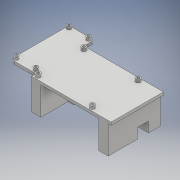
# Autodesk Inventor part: baseRaspberry
Saved by Autodesk Inventor 2018 (Build 220112000, 112)
## iProperties
Created: 2018-02-26
Part Number: baseRaspberry
Material: Genérico
Document SubType Name: Modeling
Designer: ivanb
Density: 1 g/cm^3
Appearance: Valor por defecto
Author: ivanb
## iProperties of the stored document baseRaspberry_3DPrint.ipt
Created: 2018-03-07
Part Number: baseRaspberry_3DPrint
Material: Genérico
Document SubType Name: Modeling
Designer: ivanb
Density: 1 g/cm^3
Appearance: Valor por defecto
Author: ivanb
Autodesk Inventor part; units mm, degrees
ref_plane "Plano de trabajo1" through (-77.1004, 28.9483, 0) normal (0, 0, -1) x (-1, 0, 0)
sketch "Boceto1" plane through (-77.1004, 28.9483, 0) normal (0, 0, -1) x (-1, 0, 0)
  line L0 (82, -56) -> (-3, -56)
  line L1 (-3, -56) -> (-3, 0)
  line L2 (-3, 0) -> (82, 0)
  line L3 (82, 0) -> (82, -56)
  point P0 (-77.1004, -28.9483)
  constraints: 8 end point, 2 parallel, 1 horizontal, 1 perpendicular
extrude "Extrusión1" add sketch "Boceto1" along normal blind 20
ref_plane "Plano de trabajo3" through (-77.1004, 28.9483, 0) normal (0, 0, 1) x (1, 0, 0)
sketch "Boceto2" plane through (-77.1004, 28.9483, 0) normal (0, 0, 1) x (1, 0, 0)
  circle A0 centre (-78.5, -3.5) radius 1.375 projected
  circle A1 centre (-78.5, -3.5) radius 1.125
  circle A2 centre (-20.5, -3.5) radius 1.375 projected
  circle A3 centre (-20.5, -3.5) radius 1.125
  circle A4 centre (-20.5, -52.5) radius 1.375 projected
  circle A5 centre (-20.5, -52.5) radius 1.125
  circle A6 centre (-78.5, -52.5) radius 1.375 projected
  circle A7 centre (-78.5, -52.5) radius 1.125
  line L0 (-91.1268, 5.8368) -> (25.5851, 5.8368)
  line L1 (25.5851, 5.8368) -> (25.5851, -70.6743)
  line L2 (25.5851, -70.6743) -> (-91.1268, -70.6743)
  line L3 (-91.1268, -70.6743) -> (-91.1268, 5.8368)
  point P0 (77.1004, -28.9483)
  dimension "d3" = 2.25
  dimension "d4" = 2.25
  dimension "d5" = 2.25
  dimension "d6" = 2.25
  constraints: 8 end point, 4 centre point, 4 coincident, 2 parallel, 1 horizontal, 1 perpendicular
  measures "d3" diameter of A1
  measures "d4" diameter of A3
  measures "d5" diameter of A5
  measures "d6" diameter of A7
extrude "Extrusión2" cut sketch "Boceto2" against normal blind 10 contours L0 L1 L2 L3
ref_plane "Plano de trabajo2" through (-77.1004, 28.9483, -20) normal (0, 0, -1) x (-1, 0, 0)
sketch "Boceto8" plane through (-77.1004, 28.9483, -20) normal (0, 0, -1) x (-1, 0, 0)
  circle A0 centre (77, -33) radius 1.25
  circle A1 centre (77, -5) radius 1.25
  line L0 (-3, -56) -> (82, -56) projected
  circle A2 centre (5, -33) radius 1.25
  circle A3 centre (5, -5) radius 1.25
  line L1 (82, -56) -> (82, 0) projected
  line L2 (82, -56) -> (72, -56)
  line L3 (72, -56) -> (72, 0)
  line L4 (72, 0) -> (82, 0)
  line L5 (82, 0) -> (82, -56)
  line L6 (10.1328, -56) -> (0.1328, -56)
  line L7 (5, -33) -> (5, -5)
  line L8 (0, -59.0097) -> (0, -32.6767)
  line L9 (79, -56) -> (0, -56) projected
  line L10 (0, -56) -> (10, -56)
  line L11 (10, -56) -> (10, 0)
  line L12 (10, 0) -> (0, 0)
  line L13 (0, 0) -> (0, -56)
  line L14 (82, 0) -> (-3, 0) projected
  point P0 (-77.1004, -28.9483)
  dimension "d31" = 2.5
  dimension "d32" = 2.5
  dimension "d33" = 28
  dimension "d35" = 2.5
  dimension "d36" = 72
  dimension "d37" = 2.5
  dimension "d38" = 5
  dimension "d39" = 72
  dimension "d40" = 5
  dimension "d41" = 28
  dimension "d43" = 10
  dimension "d45" = 5
  dimension "d46" = 10
  dimension "d92" = 0
  constraints: 22 end point, 4 centre point, 4 parallel, 3 horizontal, 2 perpendicular, 1 point on line, 1 vertical
  measures "d31" diameter of A0
  measures "d32" diameter of A1
  measures "d33" distance of A1.centre A0.centre
  measures "d35" diameter of A2
  measures "d36" distance of L7.start A0.centre
  measures "d37" diameter of A3
  measures "d38" distance from line of L1 A0.centre
  measures "d39" distance of L7.end A1.centre
  measures "d40" distance from line of L1 A1.centre
  measures "d41" distance of L7.end L7.start
  measures "d43" distance of L3.end L4.end
  measures "d45" distance from line of L7.start L8
  measures "d46" distance of L12.end L11.end
  measures "d92" distance between parallel lines of L14 L12
extrude "Extrusión8" add sketch "Boceto8" along normal blind 30 contours L8 L13 L12 L11 L0 | L3 L4 L1 L0
ref_plane "Plano de trabajo6" through (-159.1004, -27.0517, -10) normal (-1, 0, 0) x (0, 0, 1)
sketch "Boceto9" plane through (-159.1004, -27.0517, -10) normal (-1, 0, 0) x (0, 0, 1)
  line L0 (-29, 31) -> (-40, 31)
  line L1 (-40, 31) -> (-40, 43)
  line L2 (-40, 43) -> (-29, 43)
  line L3 (-29, 43) -> (-29, 31)
  line L4 (0, 0) -> (-40, 0) projected
  line L5 (-40, 0) -> (-40, 56) projected
  line L6 (0, 56) -> (-40, 56) projected
  point P0 (10, 27.0517)
  dimension "d49" = 11
  dimension "d50" = 12
  dimension "d52" = 0
  dimension "d82" = 13
  constraints: 8 end point, 2 parallel, 1 horizontal, 1 perpendicular
  measures "d49" distance of L1.end L2.end
  measures "d50" distance of L0.end L1.end
  measures "d52" distance between parallel lines of L5 L1
  measures "d82" distance between parallel lines of L6 L2
extrude "Extrusión9" cut sketch "Boceto9" against normal blind 100
ref_plane "Plano de trabajo5" through (-149.1004, -27.0517, -20) normal (1, 0, 0) x (0, 0, -1)
sketch "Boceto10" plane through (-149.1004, -27.0517, -20) normal (1, 0, 0) x (0, 0, -1)
  line L0 (17, 29) -> (30, 29)
  line L1 (30, 29) -> (30, 45)
  line L2 (30, 45) -> (17, 45)
  line L3 (17, 45) -> (17, 29)
  line L4 (-10, 56) -> (30, 56) projected
  line L5 (30, 31) -> (30, 0) projected
  line L6 (19, 31) -> (19, 43) projected
  line L7 (30, 31) -> (19, 31)
  line L8 (19, 31) -> (19, 43)
  line L9 (19, 43) -> (30, 43) projected
  line L10 (19, 43) -> (30, 43)
  point P0 (-20, 27.0517)
  dimension "d59" = 13
  dimension "d60" = 16
  constraints: 14 end point, 4 equal length, 2 perpendicular, 1 horizontal
  measures "d59" distance of L0.start L0.end
  measures "d60" distance of L0.end L1.end
extrude "Extrusión10" add sketch "Boceto10" along normal blind 6 contours L3 L2 L1 L9 L6 L7 L0
sketch "Boceto11" plane through (-77.1004, -27.0517, -20) normal (1, 0, 0) x (0, 0, -1)
  line L0 (30, 43) -> (30, 74)
  line L1 (17, 29) -> (30, 29)
  line L2 (30, 29) -> (30, 45)
  line L3 (30, 45) -> (17, 45)
  line L4 (17, 45) -> (17, 29)
  line L5 (30, 31) -> (19, 31)
  line L6 (19, 31) -> (30, 31)
  line L7 (30, 31) -> (19, 31)
  line L8 (19, 31) -> (19, 43)
  line L9 (19, 31) -> (19, 43)
  line L10 (30, 43) -> (19, 43)
  line L11 (19, 43) -> (30, 43)
  line L12 (19, 43) -> (30, 43) projected
  point P0 (-20, 27.0517)
  point P1 (-20, 27.0517)
  dimension "d64" = 13
  dimension "d65" = 16
  dimension "d66" = 2
  dimension "d88" = 0
  dimension "d89" = 2
  constraints: 24 end point, 3 equal length, 3 perpendicular, 1 horizontal, 1 point on line
  measures "d64" distance of L1.start L1.end
  measures "d65" distance of L1.end L2.end
  measures "d66" distance between parallel lines of L1 L5
  measures "d88" distance between parallel lines of L12 L10
  measures "d89" distance between parallel lines of L3 L10
extrude "Extrusión11" add sketch "Boceto11" against normal blind 16 contours L10 L8 L5 L2 L1 L4 L3 L0
ref_plane "Plano de trabajo4" through (-159.1004, -27.0517, -10) normal (0, -1, 0) x (1, 0, 0)
sketch "Boceto12" plane through (-159.1004, -27.0517, -10) normal (0, -1, 0) x (1, 0, 0)
  line L0 (0, 0) -> (0, -40) projected
  line L1 (0, -7) -> (97.2238, -7)
  line L2 (97.2238, -7) -> (97.2238, 2.4478)
  line L3 (97.2238, 2.4478) -> (0, 2.4478)
  line L4 (0, 2.4478) -> (0, -7)
  line L5 (72, -10) -> (10, -10) projected
  point P0 (159.1004, 10)
  dimension "d69" = 3
  constraints: 8 end point, 2 parallel, 1 horizontal, 1 perpendicular, 1 point on line
  measures "d69" distance between parallel lines of L1 L5
extrude "Extrusión12" cut sketch "Boceto12" against normal blind 60
sketch "Boceto13" plane through (-155.6004, 25.4483, 0) normal (0, 0, 1) x (1, 0, 0)
  line L0 (90.0679, 13.1573) -> (-12.4886, 13.1573)
  line L1 (-12.4886, 13.1573) -> (-12.4886, -64.4116)
  line L2 (-12.4886, -64.4116) -> (90.0679, -64.4116)
  line L3 (90.0679, -64.4116) -> (90.0679, 13.1573)
  point P0 (155.6004, -25.4483)
  constraints: 8 end point, 2 parallel, 1 horizontal, 1 perpendicular
extrude "Extrusión13" cut sketch "Boceto13" against normal blind 10
ref_plane "Plano de trabajo8" through (-159.1004, -27.0517, -17) normal (0, 0, 1) x (1, 0, 0)
sketch "Boceto14" plane through (-159.1004, -27.0517, -17) normal (0, 0, 1) x (1, 0, 0)
  circle A0 centre (61.5, 52.5) radius 1.375 projected
  circle A1 centre (61.5, 52.5) radius 1.375
  circle A2 centre (61.5, 3.5) radius 1.375 projected
  circle A3 centre (61.5, 3.5) radius 1.375
  circle A4 centre (3.5, 3.5) radius 1.375 projected
  circle A5 centre (3.5, 3.5) radius 1.375
  circle A6 centre (3.5, 52.5) radius 1.375 projected
  circle A7 centre (3.5, 52.5) radius 1.375
  point P0 (159.1004, 27.0517)
  constraints: 4 centre point, 4 coincident
extrude "Extrusión14" cut sketch "Boceto14" against normal blind 10
ref_plane "Plano de trabajo7" through (-159.1004, -27.0517, -17) normal (0, 0, 1) x (1, 0, 0)
sketch "Boceto15" plane through (-159.1004, -27.0517, -17) normal (0, 0, 1) x (1, 0, 0)
  circle A0 centre (61.5, 52.5) radius 1.375 projected
  circle A1 centre (61.5, 52.5) radius 2.5
  circle A2 centre (61.5, 3.5) radius 1.375 projected
  circle A3 centre (61.5, 3.5) radius 2.5
  circle A4 centre (3.5, 3.5) radius 1.375 projected
  circle A5 centre (3.5, 3.5) radius 2.5
  circle A6 centre (3.5, 52.5) radius 1.375 projected
  circle A7 centre (3.5, 52.5) radius 2.5
  point P0 (159.1004, 27.0517)
  dimension "d76" = 5
  dimension "d77" = 5
  dimension "d78" = 5
  dimension "d79" = 5
  constraints: 4 centre point, 4 coincident
  measures "d76" diameter of A1
  measures "d77" diameter of A3
  measures "d78" diameter of A5
  measures "d79" diameter of A7
extrude "Extrusión15" add sketch "Boceto15" along normal blind 3
sketch "Boceto16" plane through (-149.1004, -27.0517, -20) normal (0, -1, 0) x (1, 0, 0)
  line L0 (-10, 3) -> (-10, -30) projected
  line L1 (-10, 3) -> (-37, 3)
  line L2 (-37, 3) -> (-37, 0)
  line L3 (-37, 0) -> (-10, 0)
  line L4 (-10, 0) -> (-10, 3)
  point P0 (149.1004, 20)
  dimension "d93" = 27
  dimension "d94" = 3
  constraints: 8 end point, 2 parallel, 1 horizontal, 1 perpendicular
  measures "d93" distance of L3.end L2.end
  measures "d94" distance of L2.end L1.end
extrude "Extrusión16" add sketch "Boceto16" against normal blind 67
sketch "Boceto17" plane through (-74.1004, -27.0517, -17) normal (0, 0, 1) x (1, 0, 0)
  line L0 (-85.9191, 67.0002) -> (-111.9991, 67.0002)
  line L1 (-111.9991, 67.0002) -> (-111.9991, 5.5802)
  line L2 (-111.9991, 5.5802) -> (-85.9191, 5.5802)
  line L3 (-85.9191, 5.5802) -> (-85.9191, 67.0002)
  line L4 (-91.7766, 36.2902) -> (-98.9591, 36.2902)
  line L5 (-98.9591, 36.2902) -> (-98.9591, 28.1123)
  circle A0 centre (-88.4591, 64.5402) radius 1.25
  circle A1 centre (-88.4591, 8.0402) radius 1.25
  circle A2 centre (-109.4591, 64.5402) radius 1.25
  circle A3 centre (-109.4591, 8.0402) radius 1.25
  point P0 (74.1004, 27.0517)
  dimension "d97" = 26.08
  dimension "d98" = 61.42
  dimension "d99" = 2.5
  dimension "d100" = 28.25
  dimension "d101" = 10.5
  constraints: 12 end point, 4 centre point, 3 symmetric about line, 2 horizontal, 2 parallel, 1 perpendicular, 1 vertical, 5 other
  measures "d97" distance of L1.end L2.end
  measures "d98" distance of L0.end L1.end
  measures "d99" diameter of A0
  measures "d100" distance from line of L4 A0.centre
  measures "d101" distance from line of A0.centre L5
extrude "Extrusión17" cut sketch "Boceto17" against normal blind 56 contours A0 | A1 | A2 | A3
sketch "Boceto18" plane through (-74.1004, -27.0517, -17) normal (0, 0, 1) x (1, 0, 0)
  circle A0 centre (-109.4591, 64.5402) radius 1.25 projected
  circle A1 centre (-88.4591, 64.5402) radius 1.25 projected
  circle A2 centre (-88.4591, 8.0402) radius 1.25 projected
  circle A3 centre (-109.4591, 8.0402) radius 1.25 projected
  circle A4 centre (-81.5, 3.5) radius 2.5 projected
  circle A5 centre (-23.5, 52.5) radius 2.5 projected
  circle A6 centre (-23.5, 3.5) radius 2.5 projected
  circle A7 centre (-81.5, 52.5) radius 2.5 projected
  line L0 (0, 56) -> (0, 0) projected
  line L1 (-85, 56) -> (0, 56) projected
  line L2 (-85, 56) -> (-85, 67) projected
  line L3 (-112, 67) -> (-85, 67) projected
  line L4 (-112, 0) -> (-112, 67) projected
  line L5 (0, 0) -> (-112, 0) projected
  circle A8 centre (-88.4591, 64.5402) radius 2.25
  circle A9 centre (-109.4591, 64.5402) radius 2.25
  circle A10 centre (-88.4591, 8.0402) radius 2.25
  circle A11 centre (-109.4591, 8.0402) radius 2.25
  point P0 (74.1004, 27.0517)
  dimension "d104" = 5
  dimension "d105" = 4.5
  dimension "d106" = 4.5
  dimension "d107" = 4.5
  dimension "d108" = 4.5
  constraints: 4 centre point, 4 coincident
  measures "d104" diameter of A7
  measures "d105" diameter of A8
  measures "d106" diameter of A9
  measures "d107" diameter of A10
  measures "d108" diameter of A11
extrude "Extrusión18" add sketch "Boceto18" along normal blind 3 contours A8 | A9 | A10 | A11
fillet "Empalme1" radius 4 1 edges at (-186.1004, -27.0517, -18.5)
sketch "Boceto19" plane through (-74.1004, -27.0517, -17) normal (0, 0, 1) x (1, 0, 0)
  line L0 (-85, 0) -> (-85, 31) projected
  line L1 (-85, 4.711) -> (-113.131, 4.711)
  line L2 (-113.131, 4.711) -> (-113.131, -0.5367)
  line L3 (-113.131, -0.5367) -> (-85, -0.5367)
  line L4 (-85, -0.5367) -> (-85, 4.711)
  point P0 (74.1004, 27.0517)
  constraints: 8 end point, 2 parallel, 1 horizontal, 1 perpendicular, 1 point on line
extrude "Extrusión19" cut sketch "Boceto19" against normal blind 3
fillet "Empalme2" radius 4 1 edges at (-186.1004, -22.3407, -18.5)
fillet "Empalme3" radius 3 2 edges at (-159.1004, 39.9483, -18.5) (-186.1004, 39.9483, -18.5)
